Autodesk Inventor part; units mm, degrees
(part 3 of 4)
sketch "Sketch8" plane through (0, 0, 0) normal (0, -1, 0) x (1, 0, 0)
  line L0 (70.3526, -76.6897) -> (69.3526, -74.9577) projected
  line L1 (69.3526, -74.9577) -> (70.3526, -73.2256) projected
  line L2 (70.3526, -73.2256) -> (72.3526, -73.2256) projected
  line L3 (72.3526, -73.2256) -> (73.3526, -74.9577) projected
  line L4 (73.3526, -74.9577) -> (72.3526, -76.6897) projected
  line L5 (72.3526, -76.6897) -> (70.3526, -76.6897) projected
  line L6 (60.8885, -76.6897) -> (59.8885, -74.9577) projected
  line L7 (59.8885, -74.9577) -> (60.8885, -73.2256) projected
  line L8 (60.8885, -73.2256) -> (62.8885, -73.2256) projected
  line L9 (62.8885, -73.2256) -> (63.8885, -74.9577) projected
  line L10 (63.8885, -74.9577) -> (62.8885, -76.6897) projected
  line L11 (62.8885, -76.6897) -> (60.8885, -76.6897) projected
  line L12 (51.4244, -76.6897) -> (50.4244, -74.9577) projected
  line L13 (50.4244, -74.9577) -> (51.4244, -73.2256) projected
  line L14 (51.4244, -73.2256) -> (53.4244, -73.2256) projected
  line L15 (53.4244, -73.2256) -> (54.4244, -74.9577) projected
  line L16 (54.4244, -74.9577) -> (53.4244, -76.6897) projected
  line L17 (53.4244, -76.6897) -> (51.4244, -76.6897) projected
  line L18 (41.9603, -76.6897) -> (40.9603, -74.9577) projected
  line L19 (40.9603, -74.9577) -> (41.9603, -73.2256) projected
  line L20 (41.9603, -73.2256) -> (43.9603, -73.2256) projected
  line L21 (43.9603, -73.2256) -> (44.9603, -74.9577) projected
  line L22 (44.9603, -74.9577) -> (43.9603, -76.6897) projected
  line L23 (43.9603, -76.6897) -> (41.9603, -76.6897) projected
  line L24 (32.4962, -76.6897) -> (31.4962, -74.9577) projected
  line L25 (31.4962, -74.9577) -> (32.4962, -73.2256) projected
  line L26 (32.4962, -73.2256) -> (34.4962, -73.2256) projected
  line L27 (34.4962, -73.2256) -> (35.4962, -74.9577) projected
  line L28 (35.4962, -74.9577) -> (34.4962, -76.6897) projected
  line L29 (34.4962, -76.6897) -> (32.4962, -76.6897) projected
  line L30 (23.0321, -76.6897) -> (22.0321, -74.9577) projected
  line L31 (22.0321, -74.9577) -> (23.0321, -73.2256) projected
  line L32 (23.0321, -73.2256) -> (25.0321, -73.2256) projected
  line L33 (25.0321, -73.2256) -> (26.0321, -74.9577) projected
  line L34 (26.0321, -74.9577) -> (25.0321, -76.6897) projected
  line L35 (25.0321, -76.6897) -> (23.0321, -76.6897) projected
  line L36 (75.0846, -73.9577) -> (74.0846, -72.2256) projected
  line L37 (74.0846, -72.2256) -> (75.0846, -70.4936) projected
  line L38 (75.0846, -70.4936) -> (77.0846, -70.4936) projected
  line L39 (77.0846, -70.4936) -> (78.0846, -72.2256) projected
  line L40 (78.0846, -72.2256) -> (77.0846, -73.9577) projected
  line L41 (77.0846, -73.9577) -> (75.0846, -73.9577) projected
  line L42 (70.3526, -71.2256) -> (69.3526, -69.4936) projected
  line L43 (69.3526, -69.4936) -> (70.3526, -67.7615) projected
  line L44 (70.3526, -67.7615) -> (72.3526, -67.7615) projected
  line L45 (72.3526, -67.7615) -> (73.3526, -69.4936) projected
  line L46 (73.3526, -69.4936) -> (72.3526, -71.2256) projected
  line L47 (72.3526, -71.2256) -> (70.3526, -71.2256) projected
  line L48 (65.6205, -73.9577) -> (64.6205, -72.2256) projected
  line L49 (64.6205, -72.2256) -> (65.6205, -70.4936) projected
  line L50 (65.6205, -70.4936) -> (67.6205, -70.4936) projected
  line L51 (67.6205, -70.4936) -> (68.6205, -72.2256) projected
  line L52 (68.6205, -72.2256) -> (67.6205, -73.9577) projected
  line L53 (67.6205, -73.9577) -> (65.6205, -73.9577) projected
  line L54 (60.8885, -71.2256) -> (59.8885, -69.4936) projected
  line L55 (59.8885, -69.4936) -> (60.8885, -67.7615) projected
  line L56 (60.8885, -67.7615) -> (62.8885, -67.7615) projected
  line L57 (62.8885, -67.7615) -> (63.8885, -69.4936) projected
  line L58 (63.8885, -69.4936) -> (62.8885, -71.2256) projected
  line L59 (62.8885, -71.2256) -> (60.8885, -71.2256) projected
  line L60 (56.1564, -73.9577) -> (55.1564, -72.2256) projected
  line L61 (55.1564, -72.2256) -> (56.1564, -70.4936) projected
  line L62 (56.1564, -70.4936) -> (58.1564, -70.4936) projected
  line L63 (58.1564, -70.4936) -> (59.1564, -72.2256) projected
  line L64 (59.1564, -72.2256) -> (58.1564, -73.9577) projected
  line L65 (58.1564, -73.9577) -> (56.1564, -73.9577) projected
  line L66 (51.4244, -71.2256) -> (50.4244, -69.4936) projected
  line L67 (50.4244, -69.4936) -> (51.4244, -67.7615) projected
  line L68 (51.4244, -67.7615) -> (53.4244, -67.7615) projected
  line L69 (53.4244, -67.7615) -> (54.4244, -69.4936) projected
  line L70 (54.4244, -69.4936) -> (53.4244, -71.2256) projected
  line L71 (53.4244, -71.2256) -> (51.4244, -71.2256) projected
  line L72 (46.6923, -73.9577) -> (45.6923, -72.2256) projected
  line L73 (45.6923, -72.2256) -> (46.6923, -70.4936) projected
  line L74 (46.6923, -70.4936) -> (48.6923, -70.4936) projected
  line L75 (48.6923, -70.4936) -> (49.6923, -72.2256) projected
  line L76 (49.6923, -72.2256) -> (48.6923, -73.9577) projected
  line L77 (48.6923, -73.9577) -> (46.6923, -73.9577) projected
  line L78 (41.9603, -71.2256) -> (40.9603, -69.4936) projected
  line L79 (40.9603, -69.4936) -> (41.9603, -67.7615) projected
  line L80 (41.9603, -67.7615) -> (43.9603, -67.7615) projected
  line L81 (43.9603, -67.7615) -> (44.9603, -69.4936) projected
  line L82 (44.9603, -69.4936) -> (43.9603, -71.2256) projected
  line L83 (43.9603, -71.2256) -> (41.9603, -71.2256) projected
  line L84 (37.2282, -73.9577) -> (36.2282, -72.2256) projected
  line L85 (36.2282, -72.2256) -> (37.2282, -70.4936) projected
  line L86 (37.2282, -70.4936) -> (39.2282, -70.4936) projected
  line L87 (39.2282, -70.4936) -> (40.2282, -72.2256) projected
  line L88 (40.2282, -72.2256) -> (39.2282, -73.9577) projected
  line L89 (39.2282, -73.9577) -> (37.2282, -73.9577) projected
  line L90 (32.4962, -71.2256) -> (31.4962, -69.4936) projected
  line L91 (31.4962, -69.4936) -> (32.4962, -67.7615) projected
  line L92 (32.4962, -67.7615) -> (34.4962, -67.7615) projected
  line L93 (34.4962, -67.7615) -> (35.4962, -69.4936) projected
  line L94 (35.4962, -69.4936) -> (34.4962, -71.2256) projected
  line L95 (34.4962, -71.2256) -> (32.4962, -71.2256) projected
  line L96 (27.7641, -73.9577) -> (26.7641, -72.2256) projected
  line L97 (26.7641, -72.2256) -> (27.7641, -70.4936) projected
  line L98 (27.7641, -70.4936) -> (29.7641, -70.4936) projected
  line L99 (29.7641, -70.4936) -> (30.7641, -72.2256) projected
  line L100 (30.7641, -72.2256) -> (29.7641, -73.9577) projected
  line L101 (29.7641, -73.9577) -> (27.7641, -73.9577) projected
  line L102 (23.0321, -71.2256) -> (22.0321, -69.4936) projected
  line L103 (22.0321, -69.4936) -> (23.0321, -67.7615) projected
  line L104 (23.0321, -67.7615) -> (25.0321, -67.7615) projected
  line L105 (25.0321, -67.7615) -> (26.0321, -69.4936) projected
  line L106 (26.0321, -69.4936) -> (25.0321, -71.2256) projected
  line L107 (25.0321, -71.2256) -> (23.0321, -71.2256) projected
  line L108 (75.0846, -68.4936) -> (74.0846, -66.7615) projected
  line L109 (74.0846, -66.7615) -> (75.0846, -65.0295) projected
  line L110 (75.0846, -65.0295) -> (77.0846, -65.0295) projected
  line L111 (77.0846, -65.0295) -> (78.0846, -66.7615) projected
  line L112 (78.0846, -66.7615) -> (77.0846, -68.4936) projected
  line L113 (77.0846, -68.4936) -> (75.0846, -68.4936) projected
  line L114 (70.3526, -65.7615) -> (69.3526, -64.0295) projected
  line L115 (69.3526, -64.0295) -> (70.3526, -62.2974) projected
  line L116 (70.3526, -62.2974) -> (72.3526, -62.2974) projected
  line L117 (72.3526, -62.2974) -> (73.3526, -64.0295) projected
  line L118 (73.3526, -64.0295) -> (72.3526, -65.7615) projected
  line L119 (72.3526, -65.7615) -> (70.3526, -65.7615) projected
  line L120 (65.6205, -68.4936) -> (64.6205, -66.7615) projected
  line L121 (64.6205, -66.7615) -> (65.6205, -65.0295) projected
  line L122 (65.6205, -65.0295) -> (67.6205, -65.0295) projected
  line L123 (67.6205, -65.0295) -> (68.6205, -66.7615) projected
  line L124 (68.6205, -66.7615) -> (67.6205, -68.4936) projected
  line L125 (67.6205, -68.4936) -> (65.6205, -68.4936) projected
  line L126 (60.8885, -65.7615) -> (59.8885, -64.0295) projected
  line L127 (59.8885, -64.0295) -> (60.8885, -62.2974) projected
  line L128 (60.8885, -62.2974) -> (62.8885, -62.2974) projected
  line L129 (62.8885, -62.2974) -> (63.8885, -64.0295) projected
  line L130 (63.8885, -64.0295) -> (62.8885, -65.7615) projected
  line L131 (62.8885, -65.7615) -> (60.8885, -65.7615) projected
  line L132 (56.1564, -68.4936) -> (55.1564, -66.7615) projected
  line L133 (55.1564, -66.7615) -> (56.1564, -65.0295) projected
  line L134 (56.1564, -65.0295) -> (58.1564, -65.0295) projected
  line L135 (58.1564, -65.0295) -> (59.1564, -66.7615) projected
  line L136 (59.1564, -66.7615) -> (58.1564, -68.4936) projected
  line L137 (58.1564, -68.4936) -> (56.1564, -68.4936) projected
  line L138 (51.4244, -65.7615) -> (50.4244, -64.0295) projected
  line L139 (50.4244, -64.0295) -> (51.4244, -62.2974) projected
  line L140 (51.4244, -62.2974) -> (53.4244, -62.2974) projected
  line L141 (53.4244, -62.2974) -> (54.4244, -64.0295) projected
  line L142 (54.4244, -64.0295) -> (53.4244, -65.7615) projected
  line L143 (53.4244, -65.7615) -> (51.4244, -65.7615) projected
  line L144 (46.6923, -68.4936) -> (45.6923, -66.7615) projected
  line L145 (45.6923, -66.7615) -> (46.6923, -65.0295) projected
  line L146 (46.6923, -65.0295) -> (48.6923, -65.0295) projected
  line L147 (48.6923, -65.0295) -> (49.6923, -66.7615) projected
  line L148 (49.6923, -66.7615) -> (48.6923, -68.4936) projected
  line L149 (48.6923, -68.4936) -> (46.6923, -68.4936) projected
  line L150 (41.9603, -65.7615) -> (40.9603, -64.0295) projected
  line L151 (40.9603, -64.0295) -> (41.9603, -62.2974) projected
  line L152 (41.9603, -62.2974) -> (43.9603, -62.2974) projected
  line L153 (43.9603, -62.2974) -> (44.9603, -64.0295) projected
  line L154 (44.9603, -64.0295) -> (43.9603, -65.7615) projected
  line L155 (43.9603, -65.7615) -> (41.9603, -65.7615) projected
  line L156 (37.2282, -68.4936) -> (36.2282, -66.7615) projected
  line L157 (36.2282, -66.7615) -> (37.2282, -65.0295) projected
  line L158 (37.2282, -65.0295) -> (39.2282, -65.0295) projected
  line L159 (39.2282, -65.0295) -> (40.2282, -66.7615) projected
  line L160 (40.2282, -66.7615) -> (39.2282, -68.4936) projected
  line L161 (39.2282, -68.4936) -> (37.2282, -68.4936) projected
  line L162 (32.4962, -65.7615) -> (31.4962, -64.0295) projected
  line L163 (31.4962, -64.0295) -> (32.4962, -62.2974) projected
  line L164 (32.4962, -62.2974) -> (34.4962, -62.2974) projected
  line L165 (34.4962, -62.2974) -> (35.4962, -64.0295) projected
  line L166 (35.4962, -64.0295) -> (34.4962, -65.7615) projected
  line L167 (34.4962, -65.7615) -> (32.4962, -65.7615) projected
  line L168 (27.7641, -68.4936) -> (26.7641, -66.7615) projected
  line L169 (26.7641, -66.7615) -> (27.7641, -65.0295) projected
  line L170 (27.7641, -65.0295) -> (29.7641, -65.0295) projected
  line L171 (29.7641, -65.0295) -> (30.7641, -66.7615) projected
  line L172 (30.7641, -66.7615) -> (29.7641, -68.4936) projected
  line L173 (29.7641, -68.4936) -> (27.7641, -68.4936) projected
  line L174 (23.0321, -65.7615) -> (22.0321, -64.0295) projected
  line L175 (22.0321, -64.0295) -> (23.0321, -62.2974) projected
  line L176 (23.0321, -62.2974) -> (25.0321, -62.2974) projected
  line L177 (25.0321, -62.2974) -> (26.0321, -64.0295) projected
  line L178 (26.0321, -64.0295) -> (25.0321, -65.7615) projected
  line L179 (25.0321, -65.7615) -> (23.0321, -65.7615) projected
  line L180 (75.0846, -63.0295) -> (74.0846, -61.2974) projected
  line L181 (74.0846, -61.2974) -> (75.0846, -59.5654) projected
  line L182 (75.0846, -59.5654) -> (77.0846, -59.5654) projected
  line L183 (77.0846, -59.5654) -> (78.0846, -61.2974) projected
  line L184 (78.0846, -61.2974) -> (77.0846, -63.0295) projected
  line L185 (77.0846, -63.0295) -> (75.0846, -63.0295) projected
  line L186 (70.3526, -60.2974) -> (69.3526, -58.5654) projected
  line L187 (69.3526, -58.5654) -> (70.3526, -56.8333) projected
  line L188 (70.3526, -56.8333) -> (72.3526, -56.8333) projected
  line L189 (72.3526, -56.8333) -> (73.3526, -58.5654) projected
  line L190 (73.3526, -58.5654) -> (72.3526, -60.2974) projected
  line L191 (72.3526, -60.2974) -> (70.3526, -60.2974) projected
  line L192 (65.6205, -63.0295) -> (64.6205, -61.2974) projected
  line L193 (64.6205, -61.2974) -> (65.6205, -59.5654) projected
  line L194 (65.6205, -59.5654) -> (67.6205, -59.5654) projected
  line L195 (67.6205, -59.5654) -> (68.6205, -61.2974) projected
  line L196 (68.6205, -61.2974) -> (67.6205, -63.0295) projected
  line L197 (67.6205, -63.0295) -> (65.6205, -63.0295) projected
  line L198 (60.8885, -60.2974) -> (59.8885, -58.5654) projected
  line L199 (59.8885, -58.5654) -> (60.8885, -56.8333) projected
  line L200 (60.8885, -56.8333) -> (62.8885, -56.8333) projected
  line L201 (62.8885, -56.8333) -> (63.8885, -58.5654) projected
  line L202 (63.8885, -58.5654) -> (62.8885, -60.2974) projected
  line L203 (62.8885, -60.2974) -> (60.8885, -60.2974) projected
  line L204 (56.1564, -63.0295) -> (55.1564, -61.2974) projected
  line L205 (55.1564, -61.2974) -> (56.1564, -59.5654) projected
  line L206 (56.1564, -59.5654) -> (58.1564, -59.5654) projected
  line L207 (58.1564, -59.5654) -> (59.1564, -61.2974) projected
  line L208 (59.1564, -61.2974) -> (58.1564, -63.0295) projected
  line L209 (58.1564, -63.0295) -> (56.1564, -63.0295) projected
  line L210 (51.4244, -60.2974) -> (50.4244, -58.5654) projected
  line L211 (50.4244, -58.5654) -> (51.4244, -56.8333) projected
  line L212 (51.4244, -56.8333) -> (53.4244, -56.8333) projected
  line L213 (53.4244, -56.8333) -> (54.4244, -58.5654) projected
  line L214 (54.4244, -58.5654) -> (53.4244, -60.2974) projected
  line L215 (53.4244, -60.2974) -> (51.4244, -60.2974) projected
  line L216 (46.6923, -63.0295) -> (45.6923, -61.2974) projected
  line L217 (45.6923, -61.2974) -> (46.6923, -59.5654) projected
  line L218 (46.6923, -59.5654) -> (48.6923, -59.5654) projected
  line L219 (48.6923, -59.5654) -> (49.6923, -61.2974) projected
  line L220 (49.6923, -61.2974) -> (48.6923, -63.0295) projected
  line L221 (48.6923, -63.0295) -> (46.6923, -63.0295) projected
  line L222 (41.9603, -60.2974) -> (40.9603, -58.5654) projected
  line L223 (40.9603, -58.5654) -> (41.9603, -56.8333) projected
  line L224 (41.9603, -56.8333) -> (43.9603, -56.8333) projected
  line L225 (43.9603, -56.8333) -> (44.9603, -58.5654) projected
  line L226 (44.9603, -58.5654) -> (43.9603, -60.2974) projected
  line L227 (43.9603, -60.2974) -> (41.9603, -60.2974) projected
  line L228 (37.2282, -63.0295) -> (36.2282, -61.2974) projected
  line L229 (36.2282, -61.2974) -> (37.2282, -59.5654) projected
  line L230 (37.2282, -59.5654) -> (39.2282, -59.5654) projected
  line L231 (39.2282, -59.5654) -> (40.2282, -61.2974) projected
  line L232 (40.2282, -61.2974) -> (39.2282, -63.0295) projected
  line L233 (39.2282, -63.0295) -> (37.2282, -63.0295) projected
  line L234 (32.4962, -60.2974) -> (31.4962, -58.5654) projected
  line L235 (31.4962, -58.5654) -> (32.4962, -56.8333) projected
  line L236 (32.4962, -56.8333) -> (34.4962, -56.8333) projected
  line L237 (34.4962, -56.8333) -> (35.4962, -58.5654) projected
  line L238 (35.4962, -58.5654) -> (34.4962, -60.2974) projected
  line L239 (34.4962, -60.2974) -> (32.4962, -60.2974) projected
  line L240 (27.7641, -63.0295) -> (26.7641, -61.2974) projected
  line L241 (26.7641, -61.2974) -> (27.7641, -59.5654) projected
  line L242 (27.7641, -59.5654) -> (29.7641, -59.5654) projected
  line L243 (29.7641, -59.5654) -> (30.7641, -61.2974) projected
  line L244 (30.7641, -61.2974) -> (29.7641, -63.0295) projected
  line L245 (29.7641, -63.0295) -> (27.7641, -63.0295) projected
  line L246 (23.0321, -60.2974) -> (22.0321, -58.5654) projected
  line L247 (22.0321, -58.5654) -> (23.0321, -56.8333) projected
  line L248 (23.0321, -56.8333) -> (25.0321, -56.8333) projected
  line L249 (25.0321, -56.8333) -> (26.0321, -58.5654) projected
  line L250 (26.0321, -58.5654) -> (25.0321, -60.2974) projected
  line L251 (25.0321, -60.2974) -> (23.0321, -60.2974) projected
  line L252 (75.0846, -57.5654) -> (74.0846, -55.8333) projected
  line L253 (74.0846, -55.8333) -> (75.0846, -54.1013) projected
  line L254 (75.0846, -54.1013) -> (77.0846, -54.1013) projected
  line L255 (77.0846, -54.1013) -> (78.0846, -55.8333) projected
  line L256 (78.0846, -55.8333) -> (77.0846, -57.5654) projected
  line L257 (77.0846, -57.5654) -> (75.0846, -57.5654) projected
  line L258 (70.3526, -54.8333) -> (69.3526, -53.1013) projected
  line L259 (69.3526, -53.1013) -> (70.3526, -51.3692) projected
  line L260 (70.3526, -51.3692) -> (72.3526, -51.3692) projected
  line L261 (72.3526, -51.3692) -> (73.3526, -53.1013) projected
  line L262 (73.3526, -53.1013) -> (72.3526, -54.8333) projected
  line L263 (72.3526, -54.8333) -> (70.3526, -54.8333) projected
  line L264 (65.6205, -57.5654) -> (64.6205, -55.8333) projected
  line L265 (64.6205, -55.8333) -> (65.6205, -54.1013) projected
  line L266 (65.6205, -54.1013) -> (67.6205, -54.1013) projected
  line L267 (67.6205, -54.1013) -> (68.6205, -55.8333) projected
  line L268 (68.6205, -55.8333) -> (67.6205, -57.5654) projected
  line L269 (67.6205, -57.5654) -> (65.6205, -57.5654) projected
  line L270 (60.8885, -54.8333) -> (59.8885, -53.1013) projected
  line L271 (59.8885, -53.1013) -> (60.8885, -51.3692) projected
  line L272 (60.8885, -51.3692) -> (62.8885, -51.3692) projected
  line L273 (62.8885, -51.3692) -> (63.8885, -53.1013) projected
  line L274 (63.8885, -53.1013) -> (62.8885, -54.8333) projected
  line L275 (62.8885, -54.8333) -> (60.8885, -54.8333) projected
  line L276 (56.1564, -57.5654) -> (55.1564, -55.8333) projected
  line L277 (55.1564, -55.8333) -> (56.1564, -54.1013) projected
  line L278 (56.1564, -54.1013) -> (58.1564, -54.1013) projected
  line L279 (58.1564, -54.1013) -> (59.1564, -55.8333) projected
  line L280 (59.1564, -55.8333) -> (58.1564, -57.5654) projected
  line L281 (58.1564, -57.5654) -> (56.1564, -57.5654) projected
  line L282 (51.4244, -54.8333) -> (50.4244, -53.1013) projected
  line L283 (50.4244, -53.1013) -> (51.4244, -51.3692) projected
  line L284 (51.4244, -51.3692) -> (53.4244, -51.3692) projected
  line L285 (53.4244, -51.3692) -> (54.4244, -53.1013) projected
  line L286 (54.4244, -53.1013) -> (53.4244, -54.8333) projected
  line L287 (53.4244, -54.8333) -> (51.4244, -54.8333) projected
  line L288 (46.6923, -57.5654) -> (45.6923, -55.8333) projected
  line L289 (45.6923, -55.8333) -> (46.6923, -54.1013) projected
  line L290 (46.6923, -54.1013) -> (48.6923, -54.1013) projected
  line L291 (48.6923, -54.1013) -> (49.6923, -55.8333) projected
  line L292 (49.6923, -55.8333) -> (48.6923, -57.5654) projected
  line L293 (48.6923, -57.5654) -> (46.6923, -57.5654) projected
  line L294 (41.9603, -54.8333) -> (40.9603, -53.1013) projected
  line L295 (40.9603, -53.1013) -> (41.9603, -51.3692) projected
  line L296 (41.9603, -51.3692) -> (43.9603, -51.3692) projected
  line L297 (43.9603, -51.3692) -> (44.9603, -53.1013) projected
  line L298 (44.9603, -53.1013) -> (43.9603, -54.8333) projected
  line L299 (43.9603, -54.8333) -> (41.9603, -54.8333) projected
  line L300 (37.2282, -57.5654) -> (36.2282, -55.8333) projected
  line L301 (36.2282, -55.8333) -> (37.2282, -54.1013) projected
  line L302 (37.2282, -54.1013) -> (39.2282, -54.1013) projected
  line L303 (39.2282, -54.1013) -> (40.2282, -55.8333) projected
  line L304 (40.2282, -55.8333) -> (39.2282, -57.5654) projected
  line L305 (39.2282, -57.5654) -> (37.2282, -57.5654) projected
  line L306 (32.4962, -54.8333) -> (31.4962, -53.1013) projected
  line L307 (31.4962, -53.1013) -> (32.4962, -51.3692) projected
  line L308 (32.4962, -51.3692) -> (34.4962, -51.3692) projected
  line L309 (34.4962, -51.3692) -> (35.4962, -53.1013) projected
  line L310 (35.4962, -53.1013) -> (34.4962, -54.8333) projected
  line L311 (34.4962, -54.8333) -> (32.4962, -54.8333) projected
  line L312 (27.7641, -57.5654) -> (26.7641, -55.8333) projected
  line L313 (26.7641, -55.8333) -> (27.7641, -54.1013) projected
  line L314 (27.7641, -54.1013) -> (29.7641, -54.1013) projected
  line L315 (29.7641, -54.1013) -> (30.7641, -55.8333) projected
  line L316 (30.7641, -55.8333) -> (29.7641, -57.5654) projected
  line L317 (29.7641, -57.5654) -> (27.7641, -57.5654) projected
  line L318 (23.0321, -54.8333) -> (22.0321, -53.1013) projected
  line L319 (22.0321, -53.1013) -> (23.0321, -51.3692) projected
  line L320 (23.0321, -51.3692) -> (25.0321, -51.3692) projected
  line L321 (25.0321, -51.3692) -> (26.0321, -53.1013) projected
  line L322 (26.0321, -53.1013) -> (25.0321, -54.8333) projected
  line L323 (25.0321, -54.8333) -> (23.0321, -54.8333) projected
  line L324 (75.0846, -52.1013) -> (74.0846, -50.3692) projected
  line L325 (74.0846, -50.3692) -> (75.0846, -48.6372) projected
  line L326 (75.0846, -48.6372) -> (77.0846, -48.6372) projected
  line L327 (77.0846, -48.6372) -> (78.0846, -50.3692) projected
  line L328 (78.0846, -50.3692) -> (77.0846, -52.1013) projected
  line L329 (77.0846, -52.1013) -> (75.0846, -52.1013) projected
  line L330 (70.3526, -49.3692) -> (69.3526, -47.6372) projected
  line L331 (69.3526, -47.6372) -> (70.3526, -45.9051) projected
  line L332 (70.3526, -45.9051) -> (72.3526, -45.9051) projected
  line L333 (72.3526, -45.9051) -> (73.3526, -47.6372) projected
  line L334 (73.3526, -47.6372) -> (72.3526, -49.3692) projected
  line L335 (72.3526, -49.3692) -> (70.3526, -49.3692) projected
  line L336 (65.6205, -52.1013) -> (64.6205, -50.3692) projected
  line L337 (64.6205, -50.3692) -> (65.6205, -48.6372) projected
  line L338 (65.6205, -48.6372) -> (67.6205, -48.6372) projected
  line L339 (67.6205, -48.6372) -> (68.6205, -50.3692) projected
  line L340 (68.6205, -50.3692) -> (67.6205, -52.1013) projected
  line L341 (67.6205, -52.1013) -> (65.6205, -52.1013) projected
  line L342 (60.8885, -49.3692) -> (59.8885, -47.6372) projected
  line L343 (59.8885, -47.6372) -> (60.8885, -45.9051) projected
  line L344 (60.8885, -45.9051) -> (62.8885, -45.9051) projected
  line L345 (62.8885, -45.9051) -> (63.8885, -47.6372) projected
  line L346 (63.8885, -47.6372) -> (62.8885, -49.3692) projected
  line L347 (62.8885, -49.3692) -> (60.8885, -49.3692) projected
  line L348 (56.1564, -52.1013) -> (55.1564, -50.3692) projected
  line L349 (55.1564, -50.3692) -> (56.1564, -48.6372) projected
  line L350 (56.1564, -48.6372) -> (58.1564, -48.6372) projected
  line L351 (58.1564, -48.6372) -> (59.1564, -50.3692) projected
  line L352 (59.1564, -50.3692) -> (58.1564, -52.1013) projected
  line L353 (58.1564, -52.1013) -> (56.1564, -52.1013) projected
  line L354 (51.4244, -49.3692) -> (50.4244, -47.6372) projected
  line L355 (50.4244, -47.6372) -> (51.4244, -45.9051) projected
  line L356 (51.4244, -45.9051) -> (53.4244, -45.9051) projected
  line L357 (53.4244, -45.9051) -> (54.4244, -47.6372) projected
  line L358 (54.4244, -47.6372) -> (53.4244, -49.3692) projected
  line L359 (53.4244, -49.3692) -> (51.4244, -49.3692) projected
  line L360 (46.6923, -52.1013) -> (45.6923, -50.3692) projected
  line L361 (45.6923, -50.3692) -> (46.6923, -48.6372) projected
  line L362 (46.6923, -48.6372) -> (48.6923, -48.6372) projected
  line L363 (48.6923, -48.6372) -> (49.6923, -50.3692) projected
  line L364 (49.6923, -50.3692) -> (48.6923, -52.1013) projected
  line L365 (48.6923, -52.1013) -> (46.6923, -52.1013) projected
  line L366 (41.9603, -49.3692) -> (40.9603, -47.6372) projected
  line L367 (40.9603, -47.6372) -> (41.9603, -45.9051) projected
  line L368 (41.9603, -45.9051) -> (43.9603, -45.9051) projected
  line L369 (43.9603, -45.9051) -> (44.9603, -47.6372) projected
  line L370 (44.9603, -47.6372) -> (43.9603, -49.3692) projected
  line L371 (43.9603, -49.3692) -> (41.9603, -49.3692) projected
  line L372 (37.2282, -52.1013) -> (36.2282, -50.3692) projected
  line L373 (36.2282, -50.3692) -> (37.2282, -48.6372) projected
  line L374 (37.2282, -48.6372) -> (39.2282, -48.6372) projected
  line L375 (39.2282, -48.6372) -> (40.2282, -50.3692) projected
  line L376 (40.2282, -50.3692) -> (39.2282, -52.1013) projected
  line L377 (39.2282, -52.1013) -> (37.2282, -52.1013) projected
  line L378 (32.4962, -49.3692) -> (31.4962, -47.6372) projected
  line L379 (31.4962, -47.6372) -> (32.4962, -45.9051) projected
  line L380 (32.4962, -45.9051) -> (34.4962, -45.9051) projected
  line L381 (34.4962, -45.9051) -> (35.4962, -47.6372) projected
  line L382 (35.4962, -47.6372) -> (34.4962, -49.3692) projected
  line L383 (34.4962, -49.3692) -> (32.4962, -49.3692) projected
  line L384 (27.7641, -52.1013) -> (26.7641, -50.3692) projected
  line L385 (26.7641, -50.3692) -> (27.7641, -48.6372) projected
  line L386 (27.7641, -48.6372) -> (29.7641, -48.6372) projected
  line L387 (29.7641, -48.6372) -> (30.7641, -50.3692) projected
  line L388 (30.7641, -50.3692) -> (29.7641, -52.1013) projected
  line L389 (29.7641, -52.1013) -> (27.7641, -52.1013) projected
  line L390 (23.0321, -49.3692) -> (22.0321, -47.6372) projected
  line L391 (22.0321, -47.6372) -> (23.0321, -45.9051) projected
  line L392 (23.0321, -45.9051) -> (25.0321, -45.9051) projected
  line L393 (25.0321, -45.9051) -> (26.0321, -47.6372) projected
  line L394 (26.0321, -47.6372) -> (25.0321, -49.3692) projected
  line L395 (25.0321, -49.3692) -> (23.0321, -49.3692) projected
  line L396 (75.0846, -46.6372) -> (74.0846, -44.9051) projected
  line L397 (74.0846, -44.9051) -> (75.0846, -43.1731) projected
  line L398 (75.0846, -43.1731) -> (77.0846, -43.1731) projected
  line L399 (77.0846, -43.1731) -> (78.0846, -44.9051) projected
  line L400 (78.0846, -44.9051) -> (77.0846, -46.6372) projected
  line L401 (77.0846, -46.6372) -> (75.0846, -46.6372) projected
  line L402 (70.3526, -43.9051) -> (69.3526, -42.1731) projected
  line L403 (69.3526, -42.1731) -> (70.3526, -40.441) projected
  line L404 (70.3526, -40.441) -> (72.3526, -40.441) projected
  line L405 (72.3526, -40.441) -> (73.3526, -42.1731) projected
  line L406 (73.3526, -42.1731) -> (72.3526, -43.9051) projected
  line L407 (72.3526, -43.9051) -> (70.3526, -43.9051) projected
  line L408 (65.6205, -46.6372) -> (64.6205, -44.9051) projected
  line L409 (64.6205, -44.9051) -> (65.6205, -43.1731) projected
  line L410 (65.6205, -43.1731) -> (67.6205, -43.1731) projected
  line L411 (67.6205, -43.1731) -> (68.6205, -44.9051) projected
  line L412 (68.6205, -44.9051) -> (67.6205, -46.6372) projected
  line L413 (67.6205, -46.6372) -> (65.6205, -46.6372) projected
  line L414 (60.8885, -43.9051) -> (59.8885, -42.1731) projected
  line L415 (59.8885, -42.1731) -> (60.8885, -40.441) projected
  line L416 (60.8885, -40.441) -> (62.8885, -40.441) projected
  line L417 (62.8885, -40.441) -> (63.8885, -42.1731) projected
  line L418 (63.8885, -42.1731) -> (62.8885, -43.9051) projected
  line L419 (62.8885, -43.9051) -> (60.8885, -43.9051) projected
  line L420 (56.1564, -46.6372) -> (55.1564, -44.9051) projected
  line L421 (55.1564, -44.9051) -> (56.1564, -43.1731) projected
  line L422 (56.1564, -43.1731) -> (58.1564, -43.1731) projected
  line L423 (58.1564, -43.1731) -> (59.1564, -44.9051) projected
  line L424 (59.1564, -44.9051) -> (58.1564, -46.6372) projected
  line L425 (58.1564, -46.6372) -> (56.1564, -46.6372) projected
  line L426 (51.4244, -43.9051) -> (50.4244, -42.1731) projected
  line L427 (50.4244, -42.1731) -> (51.4244, -40.441) projected
  line L428 (51.4244, -40.441) -> (53.4244, -40.441) projected
  line L429 (53.4244, -40.441) -> (54.4244, -42.1731) projected
  line L430 (54.4244, -42.1731) -> (53.4244, -43.9051) projected
  line L431 (53.4244, -43.9051) -> (51.4244, -43.9051) projected
  line L432 (46.6923, -46.6372) -> (45.6923, -44.9051) projected
  line L433 (45.6923, -44.9051) -> (46.6923, -43.1731) projected
  line L434 (46.6923, -43.1731) -> (48.6923, -43.1731) projected
  line L435 (48.6923, -43.1731) -> (49.6923, -44.9051) projected
  line L436 (49.6923, -44.9051) -> (48.6923, -46.6372) projected
  line L437 (48.6923, -46.6372) -> (46.6923, -46.6372) projected
  line L438 (41.9603, -43.9051) -> (40.9603, -42.1731) projected
  line L439 (40.9603, -42.1731) -> (41.9603, -40.441) projected
  line L440 (41.9603, -40.441) -> (43.9603, -40.441) projected
  line L441 (43.9603, -40.441) -> (44.9603, -42.1731) projected
  line L442 (44.9603, -42.1731) -> (43.9603, -43.9051) projected
  line L443 (43.9603, -43.9051) -> (41.9603, -43.9051) projected
  line L444 (37.2282, -46.6372) -> (36.2282, -44.9051) projected
  line L445 (36.2282, -44.9051) -> (37.2282, -43.1731) projected
  line L446 (37.2282, -43.1731) -> (39.2282, -43.1731) projected
  line L447 (39.2282, -43.1731) -> (40.2282, -44.9051) projected
  line L448 (40.2282, -44.9051) -> (39.2282, -46.6372) projected
  line L449 (39.2282, -46.6372) -> (37.2282, -46.6372) projected
  line L450 (32.4962, -43.9051) -> (31.4962, -42.1731) projected
  line L451 (31.4962, -42.1731) -> (32.4962, -40.441) projected
  line L452 (32.4962, -40.441) -> (34.4962, -40.441) projected
  line L453 (34.4962, -40.441) -> (35.4962, -42.1731) projected
  line L454 (35.4962, -42.1731) -> (34.4962, -43.9051) projected
  line L455 (34.4962, -43.9051) -> (32.4962, -43.9051) projected
  line L456 (27.7641, -46.6372) -> (26.7641, -44.9051) projected
  line L457 (26.7641, -44.9051) -> (27.7641, -43.1731) projected
  line L458 (27.7641, -43.1731) -> (29.7641, -43.1731) projected
  line L459 (29.7641, -43.1731) -> (30.7641, -44.9051) projected
  line L460 (30.7641, -44.9051) -> (29.7641, -46.6372) projected
  line L461 (29.7641, -46.6372) -> (27.7641, -46.6372) projected
  line L462 (23.0321, -43.9051) -> (22.0321, -42.1731) projected
  line L463 (22.0321, -42.1731) -> (23.0321, -40.441) projected
  line L464 (23.0321, -40.441) -> (25.0321, -40.441) projected
  line L465 (25.0321, -40.441) -> (26.0321, -42.1731) projected
  line L466 (26.0321, -42.1731) -> (25.0321, -43.9051) projected
  line L467 (25.0321, -43.9051) -> (23.0321, -43.9051) projected
  line L468 (75.0846, -41.1731) -> (74.0846, -39.441) projected
  line L469 (74.0846, -39.441) -> (75.0846, -37.709) projected
  line L470 (75.0846, -37.709) -> (77.0846, -37.709) projected
  line L471 (77.0846, -37.709) -> (78.0846, -39.441) projected
  line L472 (78.0846, -39.441) -> (77.0846, -41.1731) projected
  line L473 (77.0846, -41.1731) -> (75.0846, -41.1731) projected
  line L474 (70.3526, -38.441) -> (69.3526, -36.709) projected
  line L475 (69.3526, -36.709) -> (70.3526, -34.9769) projected
  line L476 (70.3526, -34.9769) -> (72.3526, -34.9769) projected
  line L477 (72.3526, -34.9769) -> (73.3526, -36.709) projected
  line L478 (73.3526, -36.709) -> (72.3526, -38.441) projected
  line L479 (72.3526, -38.441) -> (70.3526, -38.441) projected
  line L480 (65.6205, -41.1731) -> (64.6205, -39.441) projected
  line L481 (64.6205, -39.441) -> (65.6205, -37.709) projected
  line L482 (65.6205, -37.709) -> (67.6205, -37.709) projected
  line L483 (67.6205, -37.709) -> (68.6205, -39.441) projected
  line L484 (68.6205, -39.441) -> (67.6205, -41.1731) projected
  line L485 (67.6205, -41.1731) -> (65.6205, -41.1731) projected
  line L486 (60.8885, -38.441) -> (59.8885, -36.709) projected
  line L487 (59.8885, -36.709) -> (60.8885, -34.9769) projected
  line L488 (60.8885, -34.9769) -> (62.8885, -34.9769) projected
  line L489 (62.8885, -34.9769) -> (63.8885, -36.709) projected
  line L490 (63.8885, -36.709) -> (62.8885, -38.441) projected
  line L491 (62.8885, -38.441) -> (60.8885, -38.441) projected
  line L492 (56.1564, -41.1731) -> (55.1564, -39.441) projected
  line L493 (55.1564, -39.441) -> (56.1564, -37.709) projected
  line L494 (56.1564, -37.709) -> (58.1564, -37.709) projected
  line L495 (58.1564, -37.709) -> (59.1564, -39.441) projected
  line L496 (59.1564, -39.441) -> (58.1564, -41.1731) projected
  line L497 (58.1564, -41.1731) -> (56.1564, -41.1731) projected
  line L498 (51.4244, -38.441) -> (50.4244, -36.709) projected
  line L499 (50.4244, -36.709) -> (51.4244, -34.9769) projected
  line L500 (51.4244, -34.9769) -> (53.4244, -34.9769) projected
  line L501 (53.4244, -34.9769) -> (54.4244, -36.709) projected
  line L502 (54.4244, -36.709) -> (53.4244, -38.441) projected
  line L503 (53.4244, -38.441) -> (51.4244, -38.441) projected
  line L504 (46.6923, -41.1731) -> (45.6923, -39.441) projected
  line L505 (45.6923, -39.441) -> (46.6923, -37.709) projected
  line L506 (46.6923, -37.709) -> (48.6923, -37.709) projected
  line L507 (48.6923, -37.709) -> (49.6923, -39.441) projected
  line L508 (49.6923, -39.441) -> (48.6923, -41.1731) projected
  line L509 (48.6923, -41.1731) -> (46.6923, -41.1731) projected
  line L510 (41.9603, -38.441) -> (40.9603, -36.709) projected
  line L511 (40.9603, -36.709) -> (41.9603, -34.9769) projected
  line L512 (41.9603, -34.9769) -> (43.9603, -34.9769) projected
  line L513 (43.9603, -34.9769) -> (44.9603, -36.709) projected
  line L514 (44.9603, -36.709) -> (43.9603, -38.441) projected
  line L515 (43.9603, -38.441) -> (41.9603, -38.441) projected
  line L516 (37.2282, -41.1731) -> (36.2282, -39.441) projected
  line L517 (36.2282, -39.441) -> (37.2282, -37.709) projected
  line L518 (37.2282, -37.709) -> (39.2282, -37.709) projected
  line L519 (39.2282, -37.709) -> (40.2282, -39.441) projected
  line L520 (40.2282, -39.441) -> (39.2282, -41.1731) projected
  line L521 (39.2282, -41.1731) -> (37.2282, -41.1731) projected
  line L522 (32.4962, -38.441) -> (31.4962, -36.709) projected
  line L523 (31.4962, -36.709) -> (32.4962, -34.9769) projected
  line L524 (32.4962, -34.9769) -> (34.4962, -34.9769) projected
  line L525 (34.4962, -34.9769) -> (35.4962, -36.709) projected
  line L526 (35.4962, -36.709) -> (34.4962, -38.441) projected
  line L527 (34.4962, -38.441) -> (32.4962, -38.441) projected
  line L528 (27.7641, -41.1731) -> (26.7641, -39.441) projected
  line L529 (26.7641, -39.441) -> (27.7641, -37.709) projected
  line L530 (27.7641, -37.709) -> (29.7641, -37.709) projected
  line L531 (29.7641, -37.709) -> (30.7641, -39.441) projected
  line L532 (30.7641, -39.441) -> (29.7641, -41.1731) projected
  line L533 (29.7641, -41.1731) -> (27.7641, -41.1731) projected
  line L534 (23.0321, -38.441) -> (22.0321, -36.709) projected
  line L535 (22.0321, -36.709) -> (23.0321, -34.9769) projected
  line L536 (23.0321, -34.9769) -> (25.0321, -34.9769) projected
  line L537 (25.0321, -34.9769) -> (26.0321, -36.709) projected
  line L538 (26.0321, -36.709) -> (25.0321, -38.441) projected
  line L539 (25.0321, -38.441) -> (23.0321, -38.441) projected
  line L540 (75.0846, -35.709) -> (74.0846, -33.9769) projected
  line L541 (74.0846, -33.9769) -> (75.0846, -32.2449) projected
  line L542 (75.0846, -32.2449) -> (77.0846, -32.2449) projected
  line L543 (77.0846, -32.2449) -> (78.0846, -33.9769) projected
  line L544 (78.0846, -33.9769) -> (77.0846, -35.709) projected
  line L545 (77.0846, -35.709) -> (75.0846, -35.709) projected
  line L546 (70.3526, -32.9769) -> (69.3526, -31.2449) projected
  line L547 (69.3526, -31.2449) -> (70.3526, -29.5128) projected
  line L548 (70.3526, -29.5128) -> (72.3526, -29.5128) projected
  line L549 (72.3526, -29.5128) -> (73.3526, -31.2449) projected
  line L550 (73.3526, -31.2449) -> (72.3526, -32.9769) projected
  line L551 (72.3526, -32.9769) -> (70.3526, -32.9769) projected
  line L552 (65.6205, -35.709) -> (64.6205, -33.9769) projected
  line L553 (64.6205, -33.9769) -> (65.6205, -32.2449) projected
  line L554 (65.6205, -32.2449) -> (67.6205, -32.2449) projected
  line L555 (67.6205, -32.2449) -> (68.6205, -33.9769) projected
  line L556 (68.6205, -33.9769) -> (67.6205, -35.709) projected
  line L557 (67.6205, -35.709) -> (65.6205, -35.709) projected
  line L558 (60.8885, -32.9769) -> (59.8885, -31.2449) projected
  line L559 (59.8885, -31.2449) -> (60.8885, -29.5128) projected
  line L560 (60.8885, -29.5128) -> (62.8885, -29.5128) projected
  line L561 (62.8885, -29.5128) -> (63.8885, -31.2449) projected
  line L562 (63.8885, -31.2449) -> (62.8885, -32.9769) projected
  line L563 (62.8885, -32.9769) -> (60.8885, -32.9769) projected
  line L564 (56.1564, -35.709) -> (55.1564, -33.9769) projected
  line L565 (55.1564, -33.9769) -> (56.1564, -32.2449) projected
  line L566 (56.1564, -32.2449) -> (58.1564, -32.2449) projected
  line L567 (58.1564, -32.2449) -> (59.1564, -33.9769) projected
  line L568 (59.1564, -33.9769) -> (58.1564, -35.709) projected
  line L569 (58.1564, -35.709) -> (56.1564, -35.709) projected
  line L570 (51.4244, -32.9769) -> (50.4244, -31.2449) projected
  line L571 (50.4244, -31.2449) -> (51.4244, -29.5128) projected
  line L572 (51.4244, -29.5128) -> (53.4244, -29.5128) projected
  line L573 (53.4244, -29.5128) -> (54.4244, -31.2449) projected
  line L574 (54.4244, -31.2449) -> (53.4244, -32.9769) projected
  line L575 (53.4244, -32.9769) -> (51.4244, -32.9769) projected
  line L576 (46.6923, -35.709) -> (45.6923, -33.9769) projected
  line L577 (45.6923, -33.9769) -> (46.6923, -32.2449) projected
  line L578 (46.6923, -32.2449) -> (48.6923, -32.2449) projected
  line L579 (48.6923, -32.2449) -> (49.6923, -33.9769) projected
  line L580 (49.6923, -33.9769) -> (48.6923, -35.709) projected
  line L581 (48.6923, -35.709) -> (46.6923, -35.709) projected
  line L582 (41.9603, -32.9769) -> (40.9603, -31.2449) projected
  line L583 (40.9603, -31.2449) -> (41.9603, -29.5128) projected
  line L584 (41.9603, -29.5128) -> (43.9603, -29.5128) projected
  line L585 (43.9603, -29.5128) -> (44.9603, -31.2449) projected
  line L586 (44.9603, -31.2449) -> (43.9603, -32.9769) projected
  line L587 (43.9603, -32.9769) -> (41.9603, -32.9769) projected
  line L588 (37.2282, -35.709) -> (36.2282, -33.9769) projected
  line L589 (36.2282, -33.9769) -> (37.2282, -32.2449) projected
  line L590 (37.2282, -32.2449) -> (39.2282, -32.2449) projected
  line L591 (39.2282, -32.2449) -> (40.2282, -33.9769) projected
  line L592 (40.2282, -33.9769) -> (39.2282, -35.709) projected
  line L593 (39.2282, -35.709) -> (37.2282, -35.709) projected
  line L594 (32.4962, -32.9769) -> (31.4962, -31.2449) projected
  line L595 (31.4962, -31.2449) -> (32.4962, -29.5128) projected
  line L596 (32.4962, -29.5128) -> (34.4962, -29.5128) projected
  line L597 (34.4962, -29.5128) -> (35.4962, -31.2449) projected
  line L598 (35.4962, -31.2449) -> (34.4962, -32.9769) projected
  line L599 (34.4962, -32.9769) -> (32.4962, -32.9769) projected
  line L600 (27.7641, -35.709) -> (26.7641, -33.9769) projected
  line L601 (26.7641, -33.9769) -> (27.7641, -32.2449) projected
  line L602 (27.7641, -32.2449) -> (29.7641, -32.2449) projected
  line L603 (29.7641, -32.2449) -> (30.7641, -33.9769) projected
  line L604 (30.7641, -33.9769) -> (29.7641, -35.709) projected
  line L605 (29.7641, -35.709) -> (27.7641, -35.709) projected
  line L606 (23.0321, -32.9769) -> (22.0321, -31.2449) projected
  line L607 (22.0321, -31.2449) -> (23.0321, -29.5128) projected
  line L608 (23.0321, -29.5128) -> (25.0321, -29.5128) projected
  line L609 (25.0321, -29.5128) -> (26.0321, -31.2449) projected
  line L610 (26.0321, -31.2449) -> (25.0321, -32.9769) projected
  line L611 (25.0321, -32.9769) -> (23.0321, -32.9769) projected
  line L612 (75.0846, -30.2449) -> (74.0846, -28.5128) projected
  line L613 (74.0846, -28.5128) -> (75.0846, -26.7808) projected
  line L614 (75.0846, -26.7808) -> (77.0846, -26.7808) projected
  line L615 (77.0846, -26.7808) -> (78.0846, -28.5128) projected
  line L616 (78.0846, -28.5128) -> (77.0846, -30.2449) projected
  line L617 (77.0846, -30.2449) -> (75.0846, -30.2449) projected
  line L618 (70.3526, -27.5128) -> (69.3526, -25.7808) projected
  line L619 (69.3526, -25.7808) -> (70.3526, -24.0487) projected
  line L620 (70.3526, -24.0487) -> (72.3526, -24.0487) projected
  line L621 (72.3526, -24.0487) -> (73.3526, -25.7808) projected
  line L622 (73.3526, -25.7808) -> (72.3526, -27.5128) projected
  line L623 (72.3526, -27.5128) -> (70.3526, -27.5128) projected
  line L624 (65.6205, -30.2449) -> (64.6205, -28.5128) projected
  line L625 (64.6205, -28.5128) -> (65.6205, -26.7808) projected
  line L626 (65.6205, -26.7808) -> (67.6205, -26.7808) projected
  line L627 (67.6205, -26.7808) -> (68.6205, -28.5128) projected
  line L628 (68.6205, -28.5128) -> (67.6205, -30.2449) projected
  line L629 (67.6205, -30.2449) -> (65.6205, -30.2449) projected
  line L630 (60.8885, -27.5128) -> (59.8885, -25.7808) projected
  line L631 (59.8885, -25.7808) -> (60.8885, -24.0487) projected
  line L632 (60.8885, -24.0487) -> (62.8885, -24.0487) projected
  line L633 (62.8885, -24.0487) -> (63.8885, -25.7808) projected
  line L634 (63.8885, -25.7808) -> (62.8885, -27.5128) projected
  line L635 (62.8885, -27.5128) -> (60.8885, -27.5128) projected
  line L636 (56.1564, -30.2449) -> (55.1564, -28.5128) projected
  line L637 (55.1564, -28.5128) -> (56.1564, -26.7808) projected
  line L638 (56.1564, -26.7808) -> (58.1564, -26.7808) projected
  line L639 (58.1564, -26.7808) -> (59.1564, -28.5128) projected
  line L640 (59.1564, -28.5128) -> (58.1564, -30.2449) projected
  line L641 (58.1564, -30.2449) -> (56.1564, -30.2449) projected
  line L642 (51.4244, -27.5128) -> (50.4244, -25.7808) projected
  line L643 (50.4244, -25.7808) -> (51.4244, -24.0487) projected
  line L644 (51.4244, -24.0487) -> (53.4244, -24.0487) projected
  line L645 (53.4244, -24.0487) -> (54.4244, -25.7808) projected
  line L646 (54.4244, -25.7808) -> (53.4244, -27.5128) projected
  line L647 (53.4244, -27.5128) -> (51.4244, -27.5128) projected
  line L648 (46.6923, -30.2449) -> (45.6923, -28.5128) projected
  line L649 (45.6923, -28.5128) -> (46.6923, -26.7808) projected
  line L650 (46.6923, -26.7808) -> (48.6923, -26.7808) projected
  line L651 (48.6923, -26.7808) -> (49.6923, -28.5128) projected
  line L652 (49.6923, -28.5128) -> (48.6923, -30.2449) projected
  line L653 (48.6923, -30.2449) -> (46.6923, -30.2449) projected
  line L654 (41.9603, -27.5128) -> (40.9603, -25.7808) projected
  line L655 (40.9603, -25.7808) -> (41.9603, -24.0487) projected
  line L656 (41.9603, -24.0487) -> (43.9603, -24.0487) projected
  line L657 (43.9603, -24.0487) -> (44.9603, -25.7808) projected
  line L658 (44.9603, -25.7808) -> (43.9603, -27.5128) projected
  line L659 (43.9603, -27.5128) -> (41.9603, -27.5128) projected
  line L660 (37.2282, -30.2449) -> (36.2282, -28.5128) projected
  line L661 (36.2282, -28.5128) -> (37.2282, -26.7808) projected
  line L662 (37.2282, -26.7808) -> (39.2282, -26.7808) projected
  line L663 (39.2282, -26.7808) -> (40.2282, -28.5128) projected
  line L664 (40.2282, -28.5128) -> (39.2282, -30.2449) projected
  line L665 (39.2282, -30.2449) -> (37.2282, -30.2449) projected
  line L666 (32.4962, -27.5128) -> (31.4962, -25.7808) projected
  line L667 (31.4962, -25.7808) -> (32.4962, -24.0487) projected
  line L668 (32.4962, -24.0487) -> (34.4962, -24.0487) projected
  line L669 (34.4962, -24.0487) -> (35.4962, -25.7808) projected
  line L670 (35.4962, -25.7808) -> (34.4962, -27.5128) projected
  line L671 (34.4962, -27.5128) -> (32.4962, -27.5128) projected
  line L672 (27.7641, -30.2449) -> (26.7641, -28.5128) projected
  line L673 (26.7641, -28.5128) -> (27.7641, -26.7808) projected
  line L674 (27.7641, -26.7808) -> (29.7641, -26.7808) projected
  line L675 (29.7641, -26.7808) -> (30.7641, -28.5128) projected
  line L676 (30.7641, -28.5128) -> (29.7641, -30.2449) projected
  line L677 (29.7641, -30.2449) -> (27.7641, -30.2449) projected
  line L678 (23.0321, -27.5128) -> (22.0321, -25.7808) projected
  line L679 (22.0321, -25.7808) -> (23.0321, -24.0487) projected
  line L680 (23.0321, -24.0487) -> (25.0321, -24.0487) projected
  line L681 (25.0321, -24.0487) -> (26.0321, -25.7808) projected
  line L682 (26.0321, -25.7808) -> (25.0321, -27.5128) projected
  line L683 (25.0321, -27.5128) -> (23.0321, -27.5128) projected
  line L684 (75.0846, -24.7808) -> (74.0846, -23.0487) projected
  line L685 (74.0846, -23.0487) -> (75.0846, -21.3167) projected
  line L686 (75.0846, -21.3167) -> (77.0846, -21.3167) projected
  line L687 (77.0846, -21.3167) -> (78.0846, -23.0487) projected
  line L688 (78.0846, -23.0487) -> (77.0846, -24.7808) projected
  line L689 (77.0846, -24.7808) -> (75.0846, -24.7808) projected
  line L690 (70.3526, -22.0487) -> (69.3526, -20.3167) projected
  line L691 (69.3526, -20.3167) -> (70.3526, -18.5846) projected
  line L692 (70.3526, -18.5846) -> (72.3526, -18.5846) projected
  line L693 (72.3526, -18.5846) -> (73.3526, -20.3167) projected
  line L694 (73.3526, -20.3167) -> (72.3526, -22.0487) projected
  line L695 (72.3526, -22.0487) -> (70.3526, -22.0487) projected
  line L696 (65.6205, -24.7808) -> (64.6205, -23.0487) projected
  line L697 (64.6205, -23.0487) -> (65.6205, -21.3167) projected
  line L698 (65.6205, -21.3167) -> (67.6205, -21.3167) projected
  line L699 (67.6205, -21.3167) -> (68.6205, -23.0487) projected
  line L700 (68.6205, -23.0487) -> (67.6205, -24.7808) projected
  line L701 (67.6205, -24.7808) -> (65.6205, -24.7808) projected
  line L702 (60.8885, -22.0487) -> (59.8885, -20.3167) projected
  line L703 (59.8885, -20.3167) -> (60.8885, -18.5846) projected
  line L704 (60.8885, -18.5846) -> (62.8885, -18.5846) projected
  line L705 (62.8885, -18.5846) -> (63.8885, -20.3167) projected
  line L706 (63.8885, -20.3167) -> (62.8885, -22.0487) projected
  line L707 (62.8885, -22.0487) -> (60.8885, -22.0487) projected
  line L708 (56.1564, -24.7808) -> (55.1564, -23.0487) projected
  line L709 (55.1564, -23.0487) -> (56.1564, -21.3167) projected
  line L710 (56.1564, -21.3167) -> (58.1564, -21.3167) projected
  line L711 (58.1564, -21.3167) -> (59.1564, -23.0487) projected
  line L712 (59.1564, -23.0487) -> (58.1564, -24.7808) projected
  line L713 (58.1564, -24.7808) -> (56.1564, -24.7808) projected
  line L714 (51.4244, -22.0487) -> (50.4244, -20.3167) projected
  line L715 (50.4244, -20.3167) -> (51.4244, -18.5846) projected
  line L716 (51.4244, -18.5846) -> (53.4244, -18.5846) projected
  line L717 (53.4244, -18.5846) -> (54.4244, -20.3167) projected
  line L718 (54.4244, -20.3167) -> (53.4244, -22.0487) projected
  line L719 (53.4244, -22.0487) -> (51.4244, -22.0487) projected
  line L720 (46.6923, -24.7808) -> (45.6923, -23.0487) projected
  line L721 (45.6923, -23.0487) -> (46.6923, -21.3167) projected
  line L722 (46.6923, -21.3167) -> (48.6923, -21.3167) projected
  line L723 (48.6923, -21.3167) -> (49.6923, -23.0487) projected
  line L724 (49.6923, -23.0487) -> (48.6923, -24.7808) projected
  line L725 (48.6923, -24.7808) -> (46.6923, -24.7808) projected
  line L726 (41.9603, -22.0487) -> (40.9603, -20.3167) projected
  line L727 (40.9603, -20.3167) -> (41.9603, -18.5846) projected
  line L728 (41.9603, -18.5846) -> (43.9603, -18.5846) projected
  line L729 (43.9603, -18.5846) -> (44.9603, -20.3167) projected
  line L730 (44.9603, -20.3167) -> (43.9603, -22.0487) projected
  line L731 (43.9603, -22.0487) -> (41.9603, -22.0487) projected
  line L732 (37.2282, -24.7808) -> (36.2282, -23.0487) projected
  line L733 (36.2282, -23.0487) -> (37.2282, -21.3167) projected
  line L734 (37.2282, -21.3167) -> (39.2282, -21.3167) projected
  line L735 (39.2282, -21.3167) -> (40.2282, -23.0487) projected
  line L736 (40.2282, -23.0487) -> (39.2282, -24.7808) projected
  line L737 (39.2282, -24.7808) -> (37.2282, -24.7808) projected
  line L738 (32.4962, -22.0487) -> (31.4962, -20.3167) projected
  line L739 (31.4962, -20.3167) -> (32.4962, -18.5846) projected
  line L740 (32.4962, -18.5846) -> (34.4962, -18.5846) projected
  line L741 (34.4962, -18.5846) -> (35.4962, -20.3167) projected
  line L742 (35.4962, -20.3167) -> (34.4962, -22.0487) projected
  line L743 (34.4962, -22.0487) -> (32.4962, -22.0487) projected
  line L744 (27.7641, -24.7808) -> (26.7641, -23.0487) projected
  line L745 (26.7641, -23.0487) -> (27.7641, -21.3167) projected
  line L746 (27.7641, -21.3167) -> (29.7641, -21.3167) projected
  line L747 (29.7641, -21.3167) -> (30.7641, -23.0487) projected
  line L748 (30.7641, -23.0487) -> (29.7641, -24.7808) projected
  line L749 (29.7641, -24.7808) -> (27.7641, -24.7808) projected
  line L750 (23.0321, -22.0487) -> (22.0321, -20.3167) projected
  line L751 (22.0321, -20.3167) -> (23.0321, -18.5846) projected
  line L752 (23.0321, -18.5846) -> (25.0321, -18.5846) projected
  line L753 (25.0321, -18.5846) -> (26.0321, -20.3167) projected
  line L754 (26.0321, -20.3167) -> (25.0321, -22.0487) projected
  line L755 (25.0321, -22.0487) -> (23.0321, -22.0487) projected
  line L756 (75.0846, -19.3167) -> (74.0846, -17.5846) projected
  line L757 (74.0846, -17.5846) -> (75.0846, -15.8526) projected
  line L758 (75.0846, -15.8526) -> (77.0846, -15.8526) projected
  line L759 (77.0846, -15.8526) -> (78.0846, -17.5846) projected
  line L760 (78.0846, -17.5846) -> (77.0846, -19.3167) projected
  line L761 (77.0846, -19.3167) -> (75.0846, -19.3167) projected
  line L762 (70.3526, -16.5846) -> (69.3526, -14.8526) projected
  line L763 (69.3526, -14.8526) -> (70.3526, -13.1205) projected
  line L764 (70.3526, -13.1205) -> (72.3526, -13.1205) projected
  line L765 (72.3526, -13.1205) -> (73.3526, -14.8526) projected
  line L766 (73.3526, -14.8526) -> (72.3526, -16.5846) projected
  line L767 (72.3526, -16.5846) -> (70.3526, -16.5846) projected
  line L768 (65.6205, -19.3167) -> (64.6205, -17.5846) projected
  line L769 (64.6205, -17.5846) -> (65.6205, -15.8526) projected
  line L770 (65.6205, -15.8526) -> (67.6205, -15.8526) projected
  line L771 (67.6205, -15.8526) -> (68.6205, -17.5846) projected
  line L772 (68.6205, -17.5846) -> (67.6205, -19.3167) projected
  line L773 (67.6205, -19.3167) -> (65.6205, -19.3167) projected
  line L774 (60.8885, -16.5846) -> (59.8885, -14.8526) projected
  line L775 (59.8885, -14.8526) -> (60.8885, -13.1205) projected
  line L776 (60.8885, -13.1205) -> (62.8885, -13.1205) projected
  line L777 (62.8885, -13.1205) -> (63.8885, -14.8526) projected
  line L778 (63.8885, -14.8526) -> (62.8885, -16.5846) projected
  line L779 (62.8885, -16.5846) -> (60.8885, -16.5846) projected
  line L780 (56.1564, -19.3167) -> (55.1564, -17.5846) projected
  line L781 (55.1564, -17.5846) -> (56.1564, -15.8526) projected
  line L782 (56.1564, -15.8526) -> (58.1564, -15.8526) projected
  line L783 (58.1564, -15.8526) -> (59.1564, -17.5846) projected
  line L784 (59.1564, -17.5846) -> (58.1564, -19.3167) projected
  line L785 (58.1564, -19.3167) -> (56.1564, -19.3167) projected
  line L786 (51.4244, -16.5846) -> (50.4244, -14.8526) projected
  line L787 (50.4244, -14.8526) -> (51.4244, -13.1205) projected
  line L788 (51.4244, -13.1205) -> (53.4244, -13.1205) projected
  line L789 (53.4244, -13.1205) -> (54.4244, -14.8526) projected
  line L790 (54.4244, -14.8526) -> (53.4244, -16.5846) projected
  line L791 (53.4244, -16.5846) -> (51.4244, -16.5846) projected
  line L792 (46.6923, -19.3167) -> (45.6923, -17.5846) projected
  line L793 (45.6923, -17.5846) -> (46.6923, -15.8526) projected
  line L794 (46.6923, -15.8526) -> (48.6923, -15.8526) projected
  line L795 (48.6923, -15.8526) -> (49.6923, -17.5846) projected
  line L796 (49.6923, -17.5846) -> (48.6923, -19.3167) projected
  line L797 (48.6923, -19.3167) -> (46.6923, -19.3167) projected
  line L798 (41.9603, -16.5846) -> (40.9603, -14.8526) projected
  line L799 (40.9603, -14.8526) -> (41.9603, -13.1205) projected
  line L800 (41.9603, -13.1205) -> (43.9603, -13.1205) projected
  line L801 (43.9603, -13.1205) -> (44.9603, -14.8526) projected
  line L802 (44.9603, -14.8526) -> (43.9603, -16.5846) projected
  line L803 (43.9603, -16.5846) -> (41.9603, -16.5846) projected
  line L804 (37.2282, -19.3167) -> (36.2282, -17.5846) projected
  line L805 (36.2282, -17.5846) -> (37.2282, -15.8526) projected
  line L806 (37.2282, -15.8526) -> (39.2282, -15.8526) projected
  line L807 (39.2282, -15.8526) -> (40.2282, -17.5846) projected
  line L808 (40.2282, -17.5846) -> (39.2282, -19.3167) projected
  line L809 (39.2282, -19.3167) -> (37.2282, -19.3167) projected
  line L810 (32.4962, -16.5846) -> (31.4962, -14.8526) projected
  line L811 (31.4962, -14.8526) -> (32.4962, -13.1205) projected
  line L812 (32.4962, -13.1205) -> (34.4962, -13.1205) projected
  line L813 (34.4962, -13.1205) -> (35.4962, -14.8526) projected
  line L814 (35.4962, -14.8526) -> (34.4962, -16.5846) projected
  line L815 (34.4962, -16.5846) -> (32.4962, -16.5846) projected
  line L816 (27.7641, -19.3167) -> (26.7641, -17.5846) projected
  line L817 (26.7641, -17.5846) -> (27.7641, -15.8526) projected
  line L818 (27.7641, -15.8526) -> (29.7641, -15.8526) projected
  line L819 (29.7641, -15.8526) -> (30.7641, -17.5846) projected
  line L820 (30.7641, -17.5846) -> (29.7641, -19.3167) projected
  line L821 (29.7641, -19.3167) -> (27.7641, -19.3167) projected
  line L822 (23.0321, -16.5846) -> (22.0321, -14.8526) projected
  line L823 (22.0321, -14.8526) -> (23.0321, -13.1205) projected
  line L824 (23.0321, -13.1205) -> (25.0321, -13.1205) projected
  line L825 (25.0321, -13.1205) -> (26.0321, -14.8526) projected
  line L826 (26.0321, -14.8526) -> (25.0321, -16.5846) projected
  line L827 (25.0321, -16.5846) -> (23.0321, -16.5846) projected
  line L828 (75.0846, -13.8526) -> (74.0846, -12.1205) projected
  line L829 (74.0846, -12.1205) -> (75.0846, -10.3885) projected
  line L830 (75.0846, -10.3885) -> (77.0846, -10.3885) projected
  line L831 (77.0846, -10.3885) -> (78.0846, -12.1205) projected
  line L832 (78.0846, -12.1205) -> (77.0846, -13.8526) projected
  line L833 (77.0846, -13.8526) -> (75.0846, -13.8526) projected
  line L834 (70.3526, -11.1205) -> (69.3526, -9.3885) projected
  line L835 (69.3526, -9.3885) -> (70.3526, -7.6564) projected
  line L836 (70.3526, -7.6564) -> (72.3526, -7.6564) projected
  line L837 (72.3526, -7.6564) -> (73.3526, -9.3885) projected
  line L838 (73.3526, -9.3885) -> (72.3526, -11.1205) projected
  line L839 (72.3526, -11.1205) -> (70.3526, -11.1205) projected
  line L840 (65.6205, -13.8526) -> (64.6205, -12.1205) projected
  line L841 (64.6205, -12.1205) -> (65.6205, -10.3885) projected
  line L842 (65.6205, -10.3885) -> (67.6205, -10.3885) projected
  line L843 (67.6205, -10.3885) -> (68.6205, -12.1205) projected
  line L844 (68.6205, -12.1205) -> (67.6205, -13.8526) projected
  line L845 (67.6205, -13.8526) -> (65.6205, -13.8526) projected
  line L846 (60.8885, -11.1205) -> (59.8885, -9.3885) projected
  line L847 (59.8885, -9.3885) -> (60.8885, -7.6564) projected
  line L848 (60.8885, -7.6564) -> (62.8885, -7.6564) projected
  line L849 (62.8885, -7.6564) -> (63.8885, -9.3885) projected
  line L850 (63.8885, -9.3885) -> (62.8885, -11.1205) projected
  line L851 (62.8885, -11.1205) -> (60.8885, -11.1205) projected
  line L852 (56.1564, -13.8526) -> (55.1564, -12.1205) projected
  line L853 (55.1564, -12.1205) -> (56.1564, -10.3885) projected
  line L854 (56.1564, -10.3885) -> (58.1564, -10.3885) projected
  line L855 (58.1564, -10.3885) -> (59.1564, -12.1205) projected
  line L856 (59.1564, -12.1205) -> (58.1564, -13.8526) projected
  line L857 (58.1564, -13.8526) -> (56.1564, -13.8526) projected
  line L858 (51.4244, -11.1205) -> (50.4244, -9.3885) projected
  line L859 (50.4244, -9.3885) -> (51.4244, -7.6564) projected
  line L860 (51.4244, -7.6564) -> (53.4244, -7.6564) projected
  line L861 (53.4244, -7.6564) -> (54.4244, -9.3885) projected
  line L862 (54.4244, -9.3885) -> (53.4244, -11.1205) projected
  line L863 (53.4244, -11.1205) -> (51.4244, -11.1205) projected
  line L864 (46.6923, -13.8526) -> (45.6923, -12.1205) projected
  line L865 (45.6923, -12.1205) -> (46.6923, -10.3885) projected
  line L866 (46.6923, -10.3885) -> (48.6923, -10.3885) projected
  line L867 (48.6923, -10.3885) -> (49.6923, -12.1205) projected
  line L868 (49.6923, -12.1205) -> (48.6923, -13.8526) projected
  line L869 (48.6923, -13.8526) -> (46.6923, -13.8526) projected
  line L870 (41.9603, -11.1205) -> (40.9603, -9.3885) projected
  line L871 (40.9603, -9.3885) -> (41.9603, -7.6564) projected
  line L872 (41.9603, -7.6564) -> (43.9603, -7.6564) projected
  line L873 (43.9603, -7.6564) -> (44.9603, -9.3885) projected
  line L874 (44.9603, -9.3885) -> (43.9603, -11.1205) projected
  line L875 (43.9603, -11.1205) -> (41.9603, -11.1205) projected
  line L876 (37.2282, -13.8526) -> (36.2282, -12.1205) projected
  line L877 (36.2282, -12.1205) -> (37.2282, -10.3885) projected
  line L878 (37.2282, -10.3885) -> (39.2282, -10.3885) projected
  line L879 (39.2282, -10.3885) -> (40.2282, -12.1205) projected
  line L880 (40.2282, -12.1205) -> (39.2282, -13.8526) projected
  line L881 (39.2282, -13.8526) -> (37.2282, -13.8526) projected
  line L882 (32.4962, -11.1205) -> (31.4962, -9.3885) projected
  line L883 (31.4962, -9.3885) -> (32.4962, -7.6564) projected
  line L884 (32.4962, -7.6564) -> (34.4962, -7.6564) projected
  line L885 (34.4962, -7.6564) -> (35.4962, -9.3885) projected
  line L886 (35.4962, -9.3885) -> (34.4962, -11.1205) projected
  line L887 (34.4962, -11.1205) -> (32.4962, -11.1205) projected
  line L888 (27.7641, -13.8526) -> (26.7641, -12.1205) projected
  line L889 (26.7641, -12.1205) -> (27.7641, -10.3885) projected
  line L890 (27.7641, -10.3885) -> (29.7641, -10.3885) projected
  line L891 (29.7641, -10.3885) -> (30.7641, -12.1205) projected
  line L892 (30.7641, -12.1205) -> (29.7641, -13.8526) projected
  line L893 (29.7641, -13.8526) -> (27.7641, -13.8526) projected
  line L894 (23.0321, -11.1205) -> (22.0321, -9.3885) projected
  line L895 (22.0321, -9.3885) -> (23.0321, -7.6564) projected
  line L896 (23.0321, -7.6564) -> (25.0321, -7.6564) projected
  line L897 (25.0321, -7.6564) -> (26.0321, -9.3885) projected
  line L898 (26.0321, -9.3885) -> (25.0321, -11.1205) projected
  line L899 (25.0321, -11.1205) -> (23.0321, -11.1205) projected
  line L900 (75.0846, -8.3885) -> (74.0846, -6.6564) projected
  line L901 (74.0846, -6.6564) -> (75.0846, -4.9244) projected
  line L902 (75.0846, -4.9244) -> (77.0846, -4.9244) projected
  line L903 (77.0846, -4.9244) -> (78.0846, -6.6564) projected
  line L904 (78.0846, -6.6564) -> (77.0846, -8.3885) projected
  line L905 (77.0846, -8.3885) -> (75.0846, -8.3885) projected
  line L906 (70.3526, -5.6564) -> (69.3526, -3.9244) projected
  line L907 (69.3526, -3.9244) -> (70.3526, -2.1923) projected
  line L908 (70.3526, -2.1923) -> (72.3526, -2.1923) projected
  line L909 (72.3526, -2.1923) -> (73.3526, -3.9244) projected
  line L910 (73.3526, -3.9244) -> (72.3526, -5.6564) projected
  line L911 (72.3526, -5.6564) -> (70.3526, -5.6564) projected